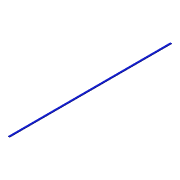
# Autodesk Inventor part: フレキラック
Saved by Autodesk Inventor 2019.4 (Build 234330000, 330)
## iProperties
Created: 2018-08-09
Part Number: フレキラック
Material: 一般
Document SubType Name: Modeling
Designer: Owner
Density: 1 g/cm^3
Appearance: 既定
Mass: 26.4 g
Surface Area: 213.46 cm^2
Volume: 26.4 cm^3
Author: Owner
Autodesk Inventor part; units mm, degrees
ref_plane "YZ Plane" through (0, 0, 0) normal (1, 0, 0) x (0, 1, 0)
ref_plane "XZ Plane" through (0, 0, 0) normal (0, 1, 0) x (-1, 0, 0)
ref_plane "XY Plane" through (0, 0, 0) normal (0, 0, 1) x (1, 0, 0)
sketch "スケッチ1" plane through (0, 0, 0) normal (0, 1, 0) x (-1, 0, 0)
  line L0 (-5, 3.3) -> (5, 3.3)
  line L1 (5, 3.3) -> (5, 0)
  line L2 (5, 0) -> (-5, 0)
  line L3 (-5, 0) -> (-5, 3.3)
  point P0 (0, 0)
  point P1 (0, 0)
  dimension "d0" = 10
  dimension "d1" = 3.3
  constraints: 8 end point, 2 parallel, 1 coincident, 1 horizontal, 1 midpoint, 1 perpendicular
  measures "d0" distance of L0.start L0.end
  measures "d1" distance of L2.end L0.start
extrude "押し出し1" add sketch "スケッチ1" along normal blind 1000
